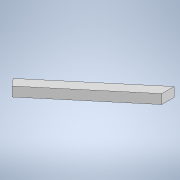
# Autodesk Inventor part: 2ndFloorOAngle
Saved by Autodesk Inventor 2020.1 (Build 241239000, 239)
## iProperties
Created: 2020-02-13
Part Number: 2ndFloorOAngle
Material: Generic
Document SubType Name: Modeling
Designer: super
Density: 1 g/cm^3
Appearance: Default
Author: super
Autodesk Inventor part; units mm, degrees
ref_plane "YZ Plane" through (0, 0, 0) normal (1, 0, 0) x (0, 1, 0)
ref_plane "XZ Plane" through (0, 0, 0) normal (0, 1, 0) x (-1, 0, 0)
ref_plane "XY Plane" through (0, 0, 0) normal (0, 0, 1) x (1, 0, 0)
sketch "Sketch1" plane through (0, 0, 0) normal (0, 1, 0) x (-1, 0, 0)
  line L0 (0, 0) -> (58.9854, 49.4946)
  line L1 (0, 0) -> (77, 0) construction
  line L2 (58.9854, 49.4946) -> (54.9037, 54.359)
  line L3 (54.9037, 54.359) -> (0, 8.2893)
  line L4 (0, 8.2893) -> (0, 0)
  dimension "d0" = 77
  dimension "d1" = 40
  dimension "d2" = 6.35
  constraints: 10 end point, 2 perpendicular, 1 equal length, 1 horizontal, 1 point on line, 1 vertical
  measures "d0" distance of L0.start L0.end
  measures "d1" angle of L1 L0
  measures "d2" distance of L0.end L2.end
extrude "Extrusion1" add sketch "Sketch1" along normal blind 6.35
body "Solid1"
